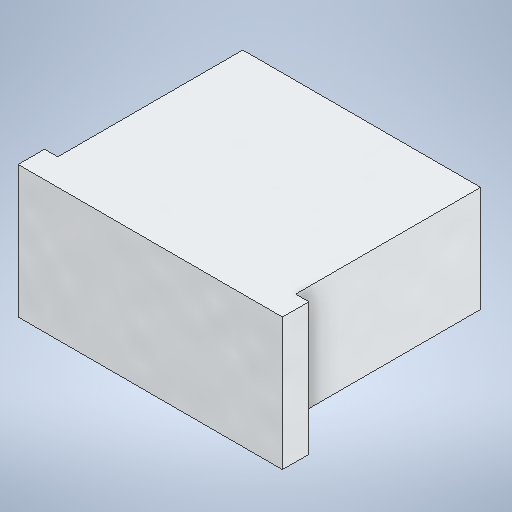
# Autodesk Inventor part: SensorPin
Saved by Autodesk Inventor 2025.1 (Build 291241020, 241B)
## iProperties
Created: 2024-09-01
Part Number: SensorPin
Material: Generic
Document SubType Name: Modeling
Designer: andre
Density: 1 g/cm^3
Appearance: Default
Author: andre
Autodesk Inventor part; units mm, degrees
ref_plane "YZ Plane" through (0, 0, 0) normal (1, 0, 0) x (0, 1, 0)
ref_plane "XZ Plane" through (0, 0, 0) normal (0, 1, 0) x (-1, 0, 0)
ref_plane "XY Plane" through (0, 0, 0) normal (0, 0, 1) x (1, 0, 0)
sketch "Sketch1" plane through (0, 0, 0) normal (0, 0, 1) x (1, 0, 0)
  line L0 (0, 0) -> (9, 0)
  line L1 (9, 0) -> (9, 4)
  line L2 (9, 4) -> (0, 4)
  line L3 (0, 4) -> (0, 0)
  dimension "d0" = 9
  dimension "d1" = 4
  constraints: 8 end point, 2 parallel, 1 horizontal, 1 perpendicular
  measures "d0" distance of L2.end L1.end
  measures "d1" distance of L1.end L0.end
extrude "Extrusion1" add sketch "Sketch1" along normal blind 7
sketch "Sketch2" plane through (0, 0, 7) normal (0, 0, 1) x (1, 0, 0)
  line L0 (-0.5, 4) -> (9.5, 4)
  line L1 (9.5, 4) -> (9.5, -1)
  line L2 (9.5, -1) -> (-0.5, -1)
  line L3 (-0.5, -1) -> (-0.5, 4)
  line L4 (9, 4) -> (0, 4) projected
  point P0 (0, 0)
  point P1 (4.5, 4)
  point P2 (4.5, 4)
  dimension "d4" = 10
  dimension "d5" = 5
  constraints: 8 end point, 2 midpoint, 2 parallel, 1 coincident, 1 horizontal, 1 horizontal alignment, 1 perpendicular
  measures "d4" distance of L0.start L0.end
  measures "d5" distance of L2.end L0.start
extrude "Extrusion2" add sketch "Sketch2" along normal blind 1
body "Solid1"
